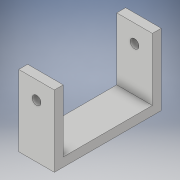
# Autodesk Inventor part: StressProngs
Saved by Autodesk Inventor 2017 (Build 210142000, 142)
## iProperties
Created: 2018-03-23
Part Number: StressProngs
Material: Generic
Document SubType Name: Modeling
Designer: User
Density: 1 g/cm^3
Appearance: Default
Author: User
Autodesk Inventor part; units mm, degrees
ref_plane "YZ Plane" through (0, 0, 0) normal (1, 0, 0) x (0, 1, 0)
ref_plane "XZ Plane" through (0, 0, 0) normal (0, 1, 0) x (-1, 0, 0)
ref_plane "XY Plane" through (0, 0, 0) normal (0, 0, 1) x (1, 0, 0)
sketch "Sketch1" plane through (0, 0, 0) normal (1, 0, 0) x (0, 1, 0)
  line L0 (0, 0) -> (50.8, 0)
  line L1 (50.8, 0) -> (50.8, -76.2)
  line L2 (50.8, -76.2) -> (0, -76.2)
  line L3 (0, -76.2) -> (0, 0)
  line L4 (50.8, -6.35) -> (6.35, -6.35)
  line L5 (6.35, -6.35) -> (6.35, -69.85)
  line L6 (6.35, -69.85) -> (50.8, -69.85)
  line L7 (50.8, -69.85) -> (50.8, -6.35)
  dimension "d0" = 50.8
  dimension "d1" = 76.2
  dimension "d2" = 6.35
  dimension "d3" = 6.35
  dimension "d4" = 6.35
  constraints: 16 end point, 4 parallel, 2 horizontal, 2 perpendicular, 1 point on line
  measures "d0" distance of L1.end L2.end
  measures "d1" distance of L0.end L1.end
  measures "d2" distance between parallel lines of L3 L5
  measures "d3" distance between parallel lines of L2 L6
  measures "d4" distance between parallel lines of L0 L4
extrude "Extrusion1" add sketch "Sketch1" along normal blind 25.4 contours L0 L1 L4 L5 L6 L2 L3
sketch "Sketch2" plane through (0, 0, 0) normal (0, 0, 1) x (1, 0, 0)
  line L0 (0, 50.8) -> (0, 0) projected
  line L1 (0, 0) -> (25.4, 0) projected
  line L2 (25.4, 50.8) -> (25.4, 0) projected
  line L3 (0, 50.8) -> (25.4, 50.8) projected
  point P0 (12.7, 38.1)
  dimension "d7" = 12.7
  dimension "d8" = 12.7
  measures "d7" distance from line of L2 point (12.7, 38.1)
  measures "d8" distance from line of L3 point (12.7, 38.1)
hole "Hole1" at (12.7, 38.1, 0) direction (0, 0, -1) diameter 6.35 end through all
body "Solid1"
